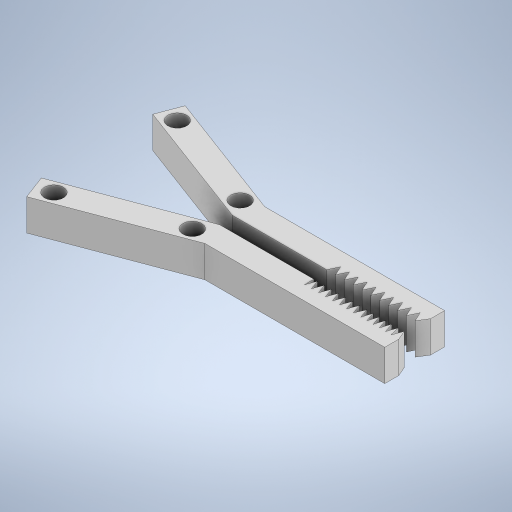
# Autodesk Inventor part: chwytakzabkikoncowka
Saved by Autodesk Inventor 2024.1 (Build 281209000, 209)
## iProperties
Created: 2023-11-11
Part Number: chwytakzabkikoncowka
Material: Generic
Document SubType Name: Modeling
Designer: Igor Sarnowski
Density: 1 g/cm^3
Appearance: Default
Author: Igor Sarnowski
Autodesk Inventor part; units mm, degrees
ref_plane "YZ Plane" through (0, 0, 0) normal (1, 0, 0) x (0, 1, 0)
ref_plane "XZ Plane" through (0, 0, 0) normal (0, 1, 0) x (-1, 0, 0)
ref_plane "XY Plane" through (0, 0, 0) normal (0, 0, 1) x (1, 0, 0)
sketch "Sketch1" plane through (0, 0, 0) normal (0, 1, 0) x (-1, 0, 0)
  line L0 (-55, -17.4998) -> (-55, -12.4998)
  line L1 (-55, -37.4998) -> (-55, -32.4998)
  circle A0 centre (-51.8947, -34.7189) radius 1.5
  circle A1 centre (-67.8947, -28.7189) radius 1.5
  circle A2 centre (-68, -20.9998) radius 1.5
  circle A3 centre (-52, -14.9998) radius 1.5
  line L2 (-49.0809, -33.638) -> (-69.3039, -26.0544)
  line L3 (-70.7084, -29.7997) -> (-50.4854, -37.3833)
  line L4 (-50.4854, -37.3833) -> (-49.0809, -33.638)
  line L5 (-49.0809, -33.638) -> (-70.7084, -29.7997) construction
  line L6 (-69.3039, -26.0544) -> (-50.4854, -37.3833) construction
  line L7 (-48.9981, -16.0101) -> (-69.5974, -23.7348)
  line L8 (-71.0019, -19.9895) -> (-50.4026, -12.2648)
  line L9 (-50.4026, -12.2648) -> (-48.9981, -16.0101)
  line L10 (-48.9981, -16.0101) -> (-71.0019, -19.9895) construction
  line L11 (-69.5974, -23.7348) -> (-50.4026, -12.2648) construction
  line L12 (-99.5974, -19.9895) -> (-71.0019, -19.9895)
  line L13 (-84.3047, -26.0571) -> (-85.0066, -27.5572)
  line L14 (-85.0066, -27.5572) -> (-85.7108, -26.0574)
  line L15 (-85.7108, -26.0574) -> (-86.4127, -27.5575)
  line L16 (-86.4127, -27.5575) -> (-87.1169, -26.0577)
  line L17 (-87.1169, -26.0577) -> (-87.8189, -27.5578)
  line L18 (-87.8189, -27.5578) -> (-88.523, -26.0579)
  line L19 (-88.523, -26.0579) -> (-89.225, -27.5581)
  line L20 (-89.225, -27.5581) -> (-89.9292, -26.0582)
  line L21 (-89.9292, -26.0582) -> (-90.6311, -27.5584)
  line L22 (-90.6311, -27.5584) -> (-91.3353, -26.0585)
  line L23 (-91.3353, -26.0585) -> (-92.0372, -27.5586)
  line L24 (-92.0372, -27.5586) -> (-92.7414, -26.0588)
  line L25 (-92.7414, -26.0588) -> (-93.4434, -27.5589)
  line L26 (-93.4434, -27.5589) -> (-94.1475, -26.059)
  line L27 (-94.1475, -26.059) -> (-94.8495, -27.5592)
  line L28 (-94.8495, -27.5592) -> (-95.5537, -26.0593)
  line L29 (-95.5537, -26.0593) -> (-96.2556, -27.5595)
  line L30 (-96.2556, -27.5595) -> (-96.9598, -26.0596)
  line L31 (-96.9598, -26.0596) -> (-97.6617, -27.5597)
  line L32 (-97.6617, -27.5597) -> (-98.3659, -26.0599)
  line L33 (-98.3659, -26.0599) -> (-99.3044, -27.5601)
  line L34 (-69.3039, -26.0544) -> (-84.3047, -26.0571)
  line L35 (-84.5974, -23.7348) -> (-84.5974, -22.2348)
  line L36 (-84.5974, -22.2348) -> (-85.1599, -23.7348)
  line L37 (-85.1599, -23.7348) -> (-85.71, -22.2348)
  line L38 (-85.71, -22.2348) -> (-86.2725, -23.7348)
  line L39 (-86.2725, -23.7348) -> (-86.8227, -22.2348)
  line L40 (-86.8227, -22.2348) -> (-87.3852, -23.7348)
  line L41 (-87.3852, -23.7348) -> (-87.9354, -22.2348)
  line L42 (-87.9354, -22.2348) -> (-88.4979, -23.7348)
  line L43 (-88.4979, -23.7348) -> (-89.0481, -22.2348)
  line L44 (-89.0481, -22.2348) -> (-89.6106, -23.7348)
  line L45 (-89.6106, -23.7348) -> (-90.1607, -22.2348)
  line L46 (-90.1607, -22.2348) -> (-90.7232, -23.7348)
  line L47 (-90.7232, -23.7348) -> (-91.2734, -22.2348)
  line L48 (-91.2734, -22.2348) -> (-91.8359, -23.7348)
  line L49 (-91.8359, -23.7348) -> (-92.3586, -22.2348)
  line L50 (-92.3586, -22.2348) -> (-93.0246, -23.7333)
  line L51 (-93.0246, -23.7333) -> (-93.5404, -22.2348)
  line L52 (-93.5404, -22.2348) -> (-94.0097, -23.7348)
  line L53 (-94.0097, -23.7348) -> (-94.526, -22.2348)
  line L54 (-94.526, -22.2348) -> (-94.9953, -23.7348)
  line L55 (-94.9953, -23.7348) -> (-95.5116, -22.2348)
  line L56 (-95.5116, -22.2348) -> (-95.9809, -23.7348)
  line L57 (-95.9809, -23.7348) -> (-96.4972, -22.2348)
  line L58 (-96.4972, -22.2348) -> (-96.9665, -23.7348)
  line L59 (-96.9665, -23.7348) -> (-97.4828, -22.2348)
  line L60 (-97.4828, -22.2348) -> (-98.0132, -23.7348)
  line L61 (-98.0132, -23.7348) -> (-98.3652, -22.2348)
  line L62 (-98.4221, -22.2348) -> (-98.9525, -23.7348)
  line L63 (-98.9525, -23.7348) -> (-99.5974, -22.2348)
  line L64 (-69.5974, -23.7348) -> (-84.5974, -23.7348)
  line L65 (-99.5974, -22.2348) -> (-99.5974, -19.9895)
  line L66 (-99.3044, -27.5601) -> (-99.3039, -29.7997)
  line L67 (-98.4221, -22.2348) -> (-98.3652, -22.2348)
  line L68 (-70.7084, -29.7997) -> (-99.3039, -29.7997)
  point P0 (0, 0)
  point P1 (-59.8947, -31.7189)
  point P2 (-60, -17.9998)
  dimension "d22" = 3
  dimension "d23" = 3
  dimension "d24" = 3
  dimension "d25" = 4
  dimension "d26" = 22
  dimension "d27" = 4
  dimension "d33" = 1.5
  constraints: 138 end point, 38 parallel, 4 centre point, 4 midpoint, 3 horizontal, 2 point on line, 1 perpendicular, 1 vertical
  measures "d22" diameter of A0
  measures "d23" diameter of A1
  measures "d24" diameter of A3
  measures "d25" distance of L3.start L2.end
  measures "d26" distance of L7.start L7.end
  measures "d27" distance of L7.end L8.start
  measures "d33" distance of L35.start L35.end
extrude "Extrusion1" add sketch "Sketch1" along normal blind 5
body "Solid1"
